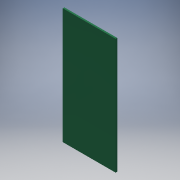
# Autodesk Inventor part: Prelim_Board
Saved by Autodesk Inventor 2016 (Build 200138000, 138)
## iProperties
Created: 2016-09-28
Part Number: Prelim_Board
Material: Generic
Document SubType Name: Modeling
Designer: jfixelle
Density: 1 g/cm^3
Appearance: Smooth - Dark Sea Green
Author: jfixelle
Autodesk Inventor part; units mm, degrees
ref_plane "YZ Plane" through (0, 0, 0) normal (1, 0, 0) x (0, 1, 0)
ref_plane "XZ Plane" through (0, 0, 0) normal (0, 1, 0) x (-1, 0, 0)
ref_plane "XY Plane" through (0, 0, 0) normal (0, 0, 1) x (1, 0, 0)
sketch "Sketch1" plane through (0, 0, 0) normal (0, 0, 1) x (1, 0, 0)
  line L0 (96.3894, 119.6934) -> (149.7294, 119.6934)
  line L1 (149.7294, 119.6934) -> (149.7294, 2.8534)
  line L2 (149.7294, 2.8534) -> (96.3894, 2.8534)
  line L3 (96.3894, 2.8534) -> (96.3894, 119.6934)
  point P0 (0, 0)
  dimension "d0" = 116.84
  dimension "d1" = 53.34
  constraints: 8 end point, 2 parallel, 1 horizontal, 1 perpendicular
  measures "d0" distance of L0.end L1.end
  measures "d1" distance of L1.end L2.end
extrude "Extrusion1" add sketch "Sketch1" along normal blind 1.6
body "Solid1"
